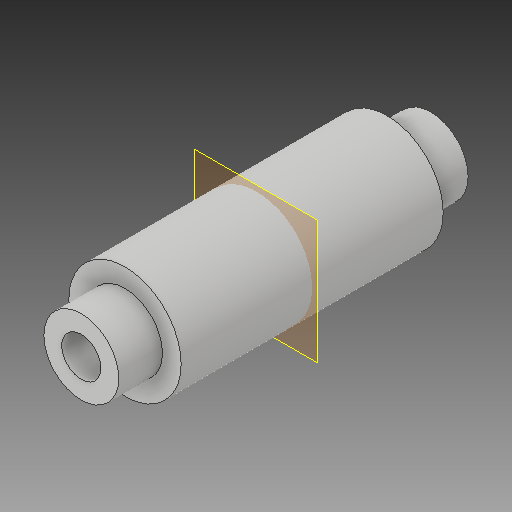
# Autodesk Inventor part: RollerSpacer2(Bearing)
Saved by Autodesk Inventor 2018 (Build 220112000, 112)
## iProperties
Created: 2020-01-25
Part Number: RollerSpacer2(Bearing)
Material: Generic
Document SubType Name: Modeling
Designer: 22jungchan
Density: 1 g/cm^3
Appearance: Default
Mass: 5.27143 g
Surface Area: 28.0582 cm^2
Volume: 5.27143 cm^3
Author: 22jungchan
Autodesk Inventor part; units mm, degrees
ref_plane "YZ Plane" through (0, 0, 0) normal (1, 0, 0) x (0, 1, 0)
ref_plane "XZ Plane" through (0, 0, 0) normal (0, 1, 0) x (-1, 0, 0)
sketch "Sketch1" plane through (0, 0, 0) normal (0, 0, 1) x (1, 0, 0)
  circle A0 centre (0, 0) radius 7.1437
  dimension "d0" = 14.2875
  constraints: 1 centre point, 1 coincident
  measures "d0" diameter of A0
extrude "Extrusion1" add sketch "Sketch1" along normal blind 33.3375
ref_plane "Work Plane1" through (0, 0, 6.35) normal (0, 0, 1) x (1, 0, 0)
sketch "Sketch6" plane through (0, 0, 33.3375) normal (0, 0, 1) x (1, 0, 0)
  circle A0 centre (0, 0) radius 2.4892
  dimension "d28" = 4.9784
  constraints: 1 centre point, 1 coincident
  measures "d28" diameter of A0
extrude "Extrusion3" cut sketch "Sketch6" against normal through all
sketch "Sketch7" plane through (0, 0, 33.3375) normal (0, 0, 1) x (1, 0, 0)
  circle A0 centre (0, 0) radius 4.7625
  circle A1 centre (0, 0) radius 2.4892
  dimension "d31" = 9.525
  dimension "d32" = 4.9784
  constraints: 2 centre point, 2 coincident
  measures "d31" diameter of A0
  measures "d32" diameter of A1
extrude "Extrusion4" add sketch "Sketch7" along normal blind 5.5563
sketch "Sketch8" plane through (0, 0, 0) normal (0, 0, -1) x (-1, 0, 0)
  circle A0 centre (0, 0) radius 2.4892 projected
  circle A1 centre (0, 0) radius 4.7625 projected
extrude "Extrusion5" add sketch "Sketch8" along normal blind 5.5563
ref_plane "Work Plane2" through (0, 0, 16.6688) normal (0, 0, 1) x (1, 0, 0)
body "Solid1"
